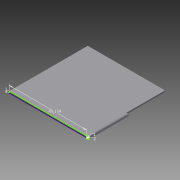
# Autodesk Inventor part: zawias
Saved by Autodesk Inventor 2014 (Build 180170000, 170)
## iProperties
Created: 2013-12-27
Part Number: zawias
Material: Ogólny
Document SubType Name: Modeling
Designer: Kuba
Density: 1 g/cm^3
Appearance: Domyślna
Author: Kuba
Autodesk Inventor part; units mm, degrees
ref_plane "YZ Plane" through (0, 0, 0) normal (1, 0, 0) x (0, 1, 0)
ref_plane "XZ Plane" through (0, 0, 0) normal (0, 1, 0) x (-1, 0, 0)
ref_plane "XY Plane" through (0, 0, 0) normal (0, 0, 1) x (1, 0, 0)
sketch "Szkic1" plane through (0, 0, 0) normal (0, 1, 0) x (-1, 0, 0)
  line L0 (0, 0) -> (-49.134, 0)
  line L1 (-49.134, 1) -> (0, 1)
  line L2 (0, 1) -> (0, 0)
  circle A0 centre (-50, 0.5) radius 1
  circle A1 centre (-50, 0.5) radius 0.5
  dimension "d2" = 2
  dimension "d3" = 1
  dimension "d4" = 49.134
  dimension "d9" = 1
  constraints: 6 end point, 2 centre point, 2 point on circle, 1 coincident, 1 horizontal, 1 parallel
  measures "d2" diameter of A0
  measures "d3" distance of L1.end L0.start
  measures "d4" distance of L1.start L1.end
  measures "d9" diameter of A1
extrude "Wyciągnięcie proste1" add sketch "Szkic1" along normal blind 50 contours L0 A0 L1 L2
extrude "Wyciągnięcie proste3" add sketch "Szkic1" along normal blind 25 contours A0
